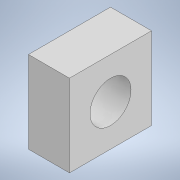
# Autodesk Inventor part: axis1
Saved by Autodesk Inventor 2022 (Build 260153000, 153)
## iProperties
Created: 2022-03-14
Part Number: axis1
Material: Generic
Document SubType Name: Modeling
Designer: br4ch
Density: 1 g/cm^3
Appearance: Default
Author: br4ch
Autodesk Inventor part; units mm, degrees
ref_plane "YZ Plane" through (0, 0, 0) normal (1, 0, 0) x (0, 1, 0)
ref_plane "XZ Plane" through (0, 0, 0) normal (0, 1, 0) x (-1, 0, 0)
ref_plane "XY Plane" through (0, 0, 0) normal (0, 0, 1) x (1, 0, 0)
sketch "Sketch1" plane through (0, 0, 0) normal (1, 0, 0) x (0, 1, 0)
  line L0 (3.5239, 5.4761) -> (-6.4761, 5.4761)
  line L1 (-6.4761, 5.4761) -> (-6.4761, -4.5239)
  line L2 (-6.4761, -4.5239) -> (3.5239, -4.5239)
  line L3 (3.5239, -4.5239) -> (3.5239, 5.4761)
  circle A0 centre (-1.4761, 0.4761) radius 2.5
  line L4 (3.5239, 5.4761) -> (-6.4761, -4.5239)
  point P0 (0, 0)
  dimension "d0" = 10
  dimension "d1" = 10
  dimension "d2" = 5
  constraints: 10 end point, 2 parallel, 1 centre point, 1 horizontal, 1 midpoint, 1 perpendicular
  measures "d0" distance of L2.end L1.end
  measures "d1" distance of L2.end L0.start
  measures "d2" diameter of A0
extrude "Extrusion1" add sketch "Sketch1" along normal blind 5 contours L4 A0 L1 L0 | L3 L2 L4 A0
body "Solid1"
